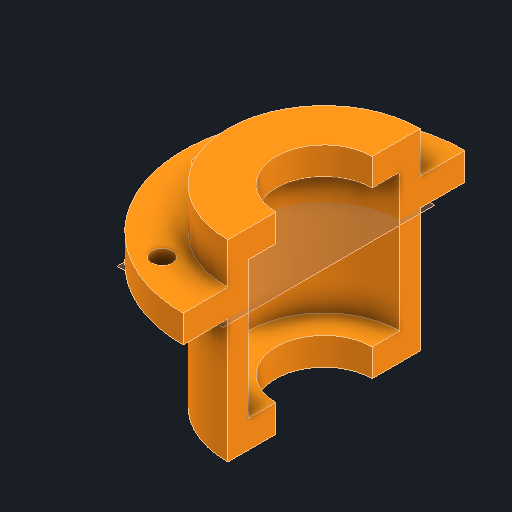
# Autodesk Inventor part: Spindle_Block_Holder
Saved by Autodesk Inventor 2024.1 (Build 281209000, 209)
## iProperties
Created: 2023-08-04
Part Number: Spindle_Block_Holder
Material: PC/ABS Plastic
Document SubType Name: Modeling
Designer: jaege
Density: 1.1 g/cm^3
Appearance: Orange
Author: jaege
Autodesk Inventor part; units mm, degrees
ref_plane "YZ Plane" through (0, 0, 0) normal (1, 0, 0) x (0, 1, 0)
ref_plane "XY Plane" through (0, 0, 0) normal (0, 0, 1) x (1, 0, 0)
sketch "Sketch1" plane through (0, 0, 0) normal (0, 1, 0) x (-1, 0, 0)
  arc A0 (0, -11) -> (0, 11) centre (0, 0) ccw
  line L0 (0, 0) -> (0, -11) construction
  line L1 (0, 0) -> (0, 11) construction
  arc A1 (0, -14) -> (0, 14) centre (0, 0) ccw
  line L2 (0, 11) -> (0, 14)
  line L3 (0, -11) -> (0, -14)
  dimension "d0" = 180
  dimension "d1" = 11
  dimension "d3" = 3
  constraints: 8 end point, 4 point on circle, 2 centre point, 2 coincident, 2 vertical, 1 collinear
  measures "d0" angle of L0 L1
  measures "d1" radius of A0
  measures "d3" distance of L2.end L1.end
extrude "Extrusion1" add sketch "Sketch1" along normal mid plane 20
sketch "Sketch2" plane through (0, 10, 0) normal (0, 1, 0) x (1, 0, 0)
  arc A0 (0, 14) -> (0, -14) centre (0, 0) ccw projected
  arc A1 (0, 11) -> (0, -11) centre (0, 0) ccw construction
  arc A2 (0, 7) -> (0, -7) centre (0, 0) ccw
  line L0 (0, 11) -> (0, 14) projected
  line L1 (0, 14) -> (0, 7)
  line L2 (0, -7) -> (0, -14)
  dimension "d6" = 4
  constraints: 4 end point, 2 collinear, 2 point on circle, 1 centre point, 1 coincident
  measures "d6" radial gap between concentric circles of A2 A1
extrude "Extrusion2" add sketch "Sketch2" along normal blind 4
sketch "Sketch3" plane through (0, -10, 0) normal (0, -1, 0) x (1, 0, 0)
  arc A0 (0, 14) -> (0, -14) centre (0, 0) ccw projected
  line L0 (0, 14) -> (0, 7) projected
  arc A1 (0, 7) -> (0, -7) centre (0, 0) ccw projected
  line L1 (0, -7) -> (0, -14) projected
  arc A2 (0, 14) -> (0, -14) centre (0, 0) ccw projected
  point P0 (0, -14)
extrude "Extrusion3" add sketch "Sketch3" along normal blind 4
ref_plane "Work Plane1" through (0, 4, 0) normal (0, 1, 0) x (-1, 0, 0)
sketch "Sketch4" plane through (0, 4, 0) normal (0, 1, 0) x (-1, 0, 0)
  arc A0 (0, -14) -> (0, 14) centre (0, 0) ccw projected
  arc A1 (0, -20.5) -> (0, 20.5) centre (0, 0) ccw
  line L0 (0, 20.5) -> (0, 14)
  line L1 (0, -14) -> (0, -20.5)
  circle A2 centre (17.25, 0) radius 1.5
  line L2 (14, 0) -> (20.5, 0) construction
  circle A3 centre (8.625, 14.9389) radius 1.5
  circle A4 centre (8.625, -14.9389) radius 1.5
  dimension "d12" = 6.5
  dimension "d13" = 3
  dimension "d16" = 60
  dimension "d20" = 60
  constraints: 6 end point, 4 centre point, 4 point on circle, 1 collinear, 1 midpoint, 1 vertical, 6 other
  measures "d12" radial gap between concentric circles of A0 A1
  measures "d13" diameter of A2
extrude "Extrusion4" add sketch "Sketch4" along normal blind 4
body "Solid1"
